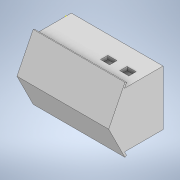
# Autodesk Inventor part: casa sip
Saved by Autodesk Inventor 2020.2 (Build 242310000, 310)
## iProperties
Created: 2020-03-20
Part Number: casa sip
Material: Generico
Document SubType Name: Modeling
Designer: kingo
Density: 1 g/cm^3
Appearance: Default
Author: kingo
Autodesk Inventor part; units mm, degrees
ref_plane "YZ Plane" through (0, 0, 0) normal (1, 0, 0) x (0, 1, 0)
ref_plane "XZ Plane" through (0, 0, 0) normal (0, 1, 0) x (-1, 0, 0)
ref_plane "XY Plane" through (0, 0, 0) normal (0, 0, 1) x (1, 0, 0)
sketch "Schizzo1" plane through (0, 0, 0) normal (0, 0, 1) x (1, 0, 0)
  line L0 (0, 0) -> (10000, 0)
  line L1 (10000, 0) -> (10000, -6000)
  line L2 (10000, -6000) -> (0, -6000)
  line L3 (0, -6000) -> (0, 0)
  line L4 (1713.9386, 0) -> (1713.9386, -400)
  line L5 (0, -1184.5275) -> (400, -1184.5275)
  line L6 (8459.3415, -6000) -> (8459.3415, -5600)
  line L7 (10000, -4879.2459) -> (9600, -4879.2459)
  line L8 (400, -400) -> (9600, -400)
  line L9 (9600, -400) -> (9600, -5600)
  line L10 (9600, -5600) -> (400, -5600)
  line L11 (400, -5600) -> (400, -400)
  dimension "d0" = 10000
  dimension "d1" = 6000
  dimension "d2" = 400
  dimension "d3" = 400
  dimension "d4" = 400
  dimension "d5" = 400
  constraints: 24 end point, 4 horizontal, 4 parallel, 4 point on line, 3 perpendicular, 1 vertical
  measures "d0" distance of L1.end L2.end
  measures "d1" distance of L0.end L1.end
  measures "d2" distance of L4.start L4.end
  measures "d3" distance of L5.start L5.end
  measures "d4" distance of L6.start L6.end
  measures "d5" distance of L7.start L7.end
extrude "Estrusione1" add sketch "Schizzo1" along normal blind 4000 contours L0 L4 L8 L11 L5 L3 | L0 L1 L7 L9 L8 L4 | L5 L11 L10 L6 L2 L3 | L1 L2 L6 L10 L9 L7
sketch "Schizzo2" plane through (0, -6000, 0) normal (0, -1, 0) x (1, 0, 0)
  line L0 (10000, 0) -> (0, 0) projected
  line L1 (6541.3712, 0) -> (6541.3712, 200)
  line L2 (6541.3712, 0) -> (6741.3712, 0) construction
  line L3 (6541.3712, 200) -> (6241.3712, 200)
  line L4 (6241.3712, 200) -> (6241.3712, 400)
  line L5 (6241.3712, 400) -> (5941.3712, 400)
  line L6 (5941.3712, 400) -> (5941.3712, 600)
  line L7 (5941.3712, 600) -> (5641.3712, 600)
  line L8 (5641.3712, 600) -> (4141.3712, 600)
  line L9 (4141.3712, 600) -> (4141.3712, 0)
  line L10 (4141.3712, 0) -> (6541.3712, 0)
  dimension "d8" = 200
  dimension "d9" = 90
  dimension "d10" = 300
  dimension "d11" = 200
  dimension "d12" = 300
  dimension "d13" = 200
  dimension "d14" = 300
  dimension "d15" = 1500
  constraints: 20 end point, 9 perpendicular, 3 point on line, 1 horizontal
  measures "d8" distance of L1.start L1.end
  measures "d9" angle of L2 L1
  measures "d10" distance of L1.end L3.end
  measures "d11" distance of L3.end L4.end
  measures "d12" distance of L4.end L5.end
  measures "d13" distance of L5.end L6.end
  measures "d14" distance of L6.end L7.end
  measures "d15" distance of L7.end L8.end
extrude "Estrusione2" add sketch "Schizzo2" along normal blind 1100
sketch "Schizzo3" plane through (0, -6000, 4000) normal (0, -1, 0) x (1, 0, 0)
  line L0 (4141.3712, -3400) -> (5941.3712, -3400) projected
  line L1 (4374.2446, -3400) -> (5574.2446, -3400)
  line L2 (5574.2446, -3400) -> (5574.2446, -1200)
  line L3 (5574.2446, -1200) -> (4374.2446, -1200)
  line L4 (4374.2446, -1200) -> (4374.2446, -3400)
  point P0 (0, -4000)
  dimension "d18" = 1200
  dimension "d19" = 2200
  constraints: 8 end point, 2 parallel, 1 horizontal, 1 perpendicular, 1 point on line
  measures "d18" distance of L3.end L2.end
  measures "d19" distance of L2.end L1.end
extrude "Estrusione3" cut sketch "Schizzo3" against normal blind 1000
sketch "Schizzo4" plane through (0, -6000, 4000) normal (0, -1, 0) x (1, 0, 0)
  line L0 (766.9374, -1200) -> (9600, -1200)
  line L1 (9600, -4000) -> (9600, 0) projected
  line L2 (1266.4462, -1200) -> (2266.4462, -1200)
  line L3 (2266.4462, -1200) -> (2266.4462, -2000)
  line L4 (2266.4462, -2000) -> (1266.4462, -2000)
  line L5 (1266.4462, -2000) -> (1266.4462, -1200)
  line L6 (5979.8517, -1200) -> (6979.8517, -1200)
  line L7 (6979.8517, -1200) -> (6979.8517, -2000)
  line L8 (6979.8517, -2000) -> (5979.8517, -2000)
  line L9 (5979.8517, -2000) -> (5979.8517, -1200)
  line L10 (8073.967, -1200) -> (9073.967, -1200)
  line L11 (9073.967, -1200) -> (9073.967, -2000)
  line L12 (9073.967, -2000) -> (8073.967, -2000)
  line L13 (8073.967, -2000) -> (8073.967, -1200)
  point P0 (0, -4000)
  dimension "d22" = 1000
  dimension "d23" = 800
  dimension "d24" = 1000
  dimension "d25" = 800
  dimension "d26" = 1000
  dimension "d27" = 800
  constraints: 26 end point, 6 parallel, 4 horizontal, 4 point on line, 3 perpendicular
  measures "d22" distance of L3.end L4.end
  measures "d23" distance of L2.end L3.end
  measures "d24" distance of L7.end L8.end
  measures "d25" distance of L6.end L7.end
  measures "d26" distance of L11.end L12.end
  measures "d27" distance of L10.end L11.end
extrude "Estrusione4" cut sketch "Schizzo4" against normal blind 1000
sketch "Schizzo5" plane through (0, 0, 0) normal (0, 1, 0) x (1, 0, 0)
  line L0 (1266.4462, -2800) -> (2266.4462, -2800) projected
  line L1 (1266.4462, -2800) -> (9246.6326, -2800)
  line L2 (8073.967, -2800) -> (9073.967, -2800) projected
  line L3 (9073.967, -2000) -> (8073.967, -2000) projected
  line L4 (9073.967, -2800) -> (8073.967, -2800)
  line L5 (8073.967, -2800) -> (8073.967, -2000)
  line L6 (8073.967, -2000) -> (9073.967, -2000)
  line L7 (9073.967, -2000) -> (9073.967, -2800)
  line L8 (6979.8517, -2800) -> (6979.8517, -2000) projected
  line L9 (5979.8517, -2000) -> (6979.8517, -2000) projected
  line L10 (6979.8517, -2800) -> (5979.8517, -2800)
  line L11 (5979.8517, -2800) -> (5979.8517, -2000)
  line L12 (5979.8517, -2000) -> (6979.8517, -2000)
  line L13 (6979.8517, -2000) -> (6979.8517, -2800)
  point P0 (0, 0)
  constraints: 18 end point, 4 parallel, 3 horizontal, 2 perpendicular
extrude "Estrusione5" cut sketch "Schizzo5" against normal blind 1000
sketch "Schizzo6" plane through (0, 0, 0) normal (0, 0, -1) x (-1, 0, 0)
  line L0 (0, -6000) -> (-10000, -6000) projected
  line L1 (-10000, -6000) -> (-10000, 0) projected
  line L2 (0, -6000) -> (-10000, -6000)
  line L3 (-10000, -6000) -> (-10000, 0)
  line L4 (-10000, 0) -> (0, 0)
  line L5 (0, 0) -> (0, -6000)
  constraints: 8 end point, 2 parallel, 1 horizontal, 1 perpendicular
extrude "Estrusione6" add sketch "Schizzo6" against normal blind 600
sketch "Schizzo7" plane through (400, -400, 600) normal (0, 0, 1) x (1, 0, 0)
  point P0 (-400, 400)
sketch "Schizzo8" plane through (0, 0, 4000) normal (0, 0, 1) x (1, 0, 0)
  line L0 (0, -6000) -> (10000, -6000) projected
  line L1 (3458.3504, -6000) -> (3458.3504, 0)
  line L2 (5574.2446, -6000) -> (5574.2446, -5600) projected
  line L3 (5574.2446, -5800) -> (5754.1703, -5800)
  line L4 (5754.1703, -5800) -> (5754.1703, 0)
  line L5 (10000, 0) -> (0, 0) projected
  line L6 (5754.1703, -5800) -> (5754.1703, -6000)
  line L7 (3458.3504, -3000) -> (0, -3000)
  line L8 (0, 0) -> (0, -6000) projected
  line L9 (9600, -400) -> (9600, -5600) projected
  line L10 (9600, -5600) -> (400, -5600) projected
  line L11 (7877.0851, -4700) -> (9600, -4700)
  line L12 (3508.3504, -6000) -> (3408.3504, -6000)
  line L13 (3408.3504, -6000) -> (3408.3504, 0)
  line L14 (3408.3504, 0) -> (3508.3504, 0)
  line L15 (3508.3504, 0) -> (3508.3504, -6000)
  line L16 (3508.3504, -6000) -> (3408.3504, 0) construction
  line L17 (3408.3504, -6000) -> (3508.3504, 0) construction
  line L18 (-50, -3050) -> (-50, -2950)
  line L19 (-50, -2950) -> (3508.3504, -2950)
  line L20 (3508.3504, -2950) -> (3508.3504, -3050)
  line L21 (3508.3504, -3050) -> (-50, -3050)
  line L22 (-50, -3050) -> (3508.3504, -2950) construction
  line L23 (-50, -2950) -> (3508.3504, -3050) construction
  line L24 (5804.1703, -5800) -> (5704.1703, -5800)
  line L25 (5704.1703, -5800) -> (5704.1703, 0)
  line L26 (5704.1703, 0) -> (5804.1703, 0)
  line L27 (5804.1703, 0) -> (5804.1703, -5800)
  line L28 (5804.1703, -5800) -> (5704.1703, 0) construction
  line L29 (5704.1703, -5800) -> (5804.1703, 0) construction
  line L30 (5804.1703, -5800) -> (5904.1703, -5800) construction
  line L31 (9600, -4750) -> (9600, -4650)
  line L32 (9600, -4650) -> (7877.0851, -4650)
  line L33 (7877.0851, -4650) -> (7877.0851, -4750)
  line L34 (7877.0851, -4750) -> (9600, -4750)
  line L35 (9600, -4750) -> (7877.0851, -4650) construction
  line L36 (9600, -4650) -> (7877.0851, -4750) construction
  line L37 (7877.0851, 0) -> (7877.0851, -4750)
  line L38 (7927.0851, -4750) -> (7827.0851, -4750)
  line L39 (7827.0851, -4750) -> (7827.0851, 0)
  line L40 (7827.0851, 0) -> (7927.0851, 0)
  line L41 (7927.0851, 0) -> (7927.0851, -4750)
  line L42 (7927.0851, -4750) -> (7827.0851, 0) construction
  line L43 (7827.0851, -4750) -> (7927.0851, 0) construction
  point P0 (1729.1752, -3000)
  point P1 (5754.1703, -2900)
  point P2 (8738.5426, -4700)
  point P3 (7877.0851, -2375)
  point P4 (7927.0851, -4650)
  point P5 (3408.3504, -3050)
  point P6 (3408.3504, -2950)
  dimension "d35" = 100
  dimension "d36" = 100
  dimension "d37" = 100
  dimension "d38" = 180
  dimension "d39" = 100
  dimension "d40" = 100
  constraints: 76 end point, 17 midpoint, 12 perpendicular, 10 parallel, 5 point on line, 2 horizontal, 2 vertical, 1 collinear
  measures "d35" distance of L12.start L12.end
  measures "d36" distance of L18.start L18.end
  measures "d37" distance of L24.start L24.end
  measures "d38" angle of L24 L30
  measures "d39" distance of L31.start L31.end
  measures "d40" distance of L38.start L38.end
extrude "Estrusione7" add sketch "Schizzo8" against normal blind 4000 contours L13 L10 L1 L0 | L21 L18 L19 L8 | L8 L7 L13 L21 | L1 L10 L15 L0 | L13 L21 L1 L10 | L8 L19 L13 L7 | L13 L7 L1 L21 | L1 L21 L15 L10 | L13 L19 L1 L7 | L1 L19 L15 L21 | L13 L5 L1 L19 | L1 L5 L15 L19 | L3 L25 L10 L4 | L4 L10 L27 L24 | L25 L5 L4 L10 | L4 L5 L27 L10 | L5 L37 L33 L38 L39 | L34 L41 L11 L9 | L5 L41 L32 L37 | L11 L41 L32 L9 | L34 L33 L11 L41 | L32 L41 L11 L33
sketch "Schizzo9" plane through (0, 0, 4000) normal (0, 0, 1) x (1, 0, 0)
  line L0 (0, -3050) -> (-50, -3050) projected
  line L1 (0, -2950) -> (-50, -2950) projected
  line L2 (-50, -3050) -> (0, -3050)
  line L3 (0, -3050) -> (0, -2950)
  line L4 (0, -2950) -> (-50, -2950)
  line L5 (-50, -2950) -> (-50, -3050)
  point P0 (0, 0)
  constraints: 8 end point, 2 parallel, 1 horizontal, 1 perpendicular
extrude "Estrusione8" cut sketch "Schizzo9" against normal blind 4000
sketch "Schizzo10" plane through (3508.3504, -5600, 4000) normal (1, 0, 0) x (0, 0, -1)
  line L0 (3400, 0) -> (3400, 2550) projected
  line L1 (3400, 2550) -> (3400, 2250)
  line L2 (3400, 5200) -> (3400, 0) projected
  line L3 (3400, 2250) -> (1300, 2250)
  line L4 (3400, 2250) -> (5500, 2250) construction
  line L5 (1300, 2250) -> (1300, 1450)
  line L6 (1300, 1450) -> (3400, 1450)
  line L7 (3400, 2250) -> (3400, 1450)
  line L8 (0, 2650) -> (3400, 2650) projected
  line L9 (3400, 2650) -> (3400, 2950)
  line L10 (3400, 2950) -> (1300, 2950)
  line L11 (1300, 2950) -> (1300, 3750)
  line L12 (1300, 3750) -> (3400, 3750)
  line L13 (3400, 2950) -> (3400, 3750)
  point P0 (4000, 5600)
  dimension "d45" = 300
  dimension "d46" = 2100
  dimension "d47" = 180
  dimension "d48" = 800
  dimension "d49" = 300
  dimension "d50" = 800
  dimension "d51" = 90
  constraints: 22 end point, 6 perpendicular, 5 point on line, 3 collinear, 1 horizontal
  measures "d45" distance of L0.end L1.end
  measures "d46" distance of L1.end L3.end
  measures "d47" angle of L3 L4
  measures "d48" distance of L3.end L5.end
  measures "d49" distance of L8.end L9.end
  measures "d50" distance of L10.end L11.end
  measures "d51" angle of L10 L11
extrude "Estrusione9" cut sketch "Schizzo10" against normal blind 1000
sketch "Schizzo11" plane through (5704.1703, -5600, 4000) normal (-1, 0, 0) x (0, 0, 1)
  line L0 (-3400, 0) -> (-3400, 5200) projected
  line L1 (-3400, 0) -> (-3400, 300)
  line L2 (-3400, 300) -> (-1300, 300)
  line L3 (-1300, 300) -> (-1300, 1100)
  line L4 (-1300, 1100) -> (-3400, 1100)
  line L5 (-3400, 5200) -> (-3400, 0) projected
  line L6 (-3400, 1100) -> (-3400, 300)
  point P0 (-4000, 5600)
  dimension "d54" = 300
  dimension "d55" = 2100
  dimension "d56" = 90
  dimension "d57" = 800
  dimension "d58" = 2100
  dimension "d59" = 90
  constraints: 10 end point, 3 perpendicular, 1 point on line
  measures "d54" distance of L0.start L1.end
  measures "d55" distance of L1.end L2.end
  measures "d56" angle of L1 L2
  measures "d57" distance of L2.end L3.end
  measures "d58" distance of L3.end L4.end
  measures "d59" angle of L4 L3
extrude "Estrusione10" cut sketch "Schizzo11" against normal blind 1000
sketch "Schizzo12" plane through (7827.0851, -4750, 4000) normal (0, -1, 0) x (1, 0, 0)
  line L0 (0, 0) -> (1772.9149, 0) projected
  line L1 (886.4574, 0) -> (886.4574, -3400)
  line L2 (1772.9149, -3400) -> (0, -3400) projected
  line L3 (886.4574, -3400) -> (1286.4574, -3400)
  line L4 (1286.4574, -3400) -> (1286.4574, -1300)
  line L5 (1286.4574, -1300) -> (486.4574, -1300)
  line L6 (486.4574, -1300) -> (486.4574, -3400)
  line L7 (486.4574, -3400) -> (1286.4574, -3400)
  point P0 (-7827.0851, -4000)
  dimension "d62" = 400
  dimension "d63" = 2100
  dimension "d64" = 90
  dimension "d65" = 800
  dimension "d66" = 90
  dimension "d67" = 2100
  dimension "d68" = 90
  constraints: 12 end point, 4 perpendicular, 2 midpoint
  measures "d62" distance of L1.end L3.end
  measures "d63" distance of L3.end L4.end
  measures "d64" angle of L4 L3
  measures "d65" distance of L4.end L5.end
  measures "d66" angle of L5 L4
  measures "d67" distance of L5.end L6.end
  measures "d68" angle of L6 L5
extrude "Estrusione11" cut sketch "Schizzo12" against normal blind 1000
sketch "Schizzo13" plane through (0, 0, 4000) normal (0, 0, 1) x (1, 0, 0)
  line L0 (10000, 0) -> (0, 0) projected
  line L1 (0, -6000) -> (10000, -6000) projected
  line L2 (0, 0) -> (10000, 0)
  line L3 (10000, 0) -> (10000, -6000)
  line L4 (10000, -6000) -> (0, -6000)
  line L5 (0, -6000) -> (0, 0)
  constraints: 8 end point, 2 parallel, 1 horizontal, 1 perpendicular
extrude "Estrusione12" add sketch "Schizzo13" along normal blind 200
sketch "Schizzo14" plane through (10000, -6000, 0) normal (1, 0, 0) x (0, 0, -1)
  line L0 (-4200, 0) -> (-4200, 6000) projected
  line L1 (-4200, 3000) -> (-5700, 3000)
  line L2 (0, 0) -> (-4200, 0) projected
  line L3 (-5700, 3000) -> (-4200, 0)
  line L4 (-4200, 0) -> (-3976.3932, -447.2136)
  line L5 (-3976.3932, -447.2136) -> (-4155.2786, -536.6563)
  line L6 (-4155.2786, -536.6563) -> (-5923.6068, 3000)
  line L7 (-5700, 3000) -> (-4200, 6000)
  line L8 (0, 6000) -> (-4200, 6000) projected
  line L9 (-4200, 0) -> (-4200, 6000)
  line L10 (-4352.4612, 5695.0777) -> (-3975.4575, 6449.0849)
  line L11 (-3975.4575, 6449.0849) -> (-4154.343, 6538.5277)
  line L12 (-4154.343, 6538.5277) -> (-5923.6068, 3000)
  dimension "d73" = 1500
  dimension "d74" = 500
  dimension "d75" = 200
  dimension "d78" = 200
  constraints: 20 end point, 3 point on line, 1 horizontal, 1 midpoint, 1 parallel, 1 perpendicular, 1 vertical
  measures "d73" distance of L1.start L1.end
  measures "d74" distance of L0.start L4.end
  measures "d75" distance of L4.end L5.end
  measures "d78" distance of L10.end L11.end
extrude "Estrusione13" add sketch "Schizzo14" against normal blind 10000
